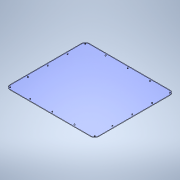
# Autodesk Inventor part: right_pane_outerl
Saved by Autodesk Inventor 2022 (Build 260153000, 153)
## iProperties
Created: 2021-05-16
Part Number: right_pane_outerl
Material: Generic
Document SubType Name: Modeling
Designer: gisen
Density: 1 g/cm^3
Appearance: Clear - Blue
Author: gisen
Autodesk Inventor part; units mm, degrees
ref_plane "YZ Plane" through (0, 0, 0) normal (1, 0, 0) x (0, 1, 0)
ref_plane "XZ Plane" through (0, 0, 0) normal (0, 1, 0) x (-1, 0, 0)
ref_plane "XY Plane" through (0, 0, 0) normal (0, 0, 1) x (1, 0, 0)
sketch "Sketch1" plane through (0, 0, 0) normal (0, 0, 1) x (1, 0, 0)
  line L0 (-196.0353, 191.75) -> (194.1012, 191.75)
  line L1 (213.9647, 171.6135) -> (213.9647, -172.019)
  line L2 (193.2337, -192.75) -> (-195.7732, -192.75)
  line L3 (-216.0353, -173.0121) -> (-216.0353, 171.75)
  line L4 (-205, 191.75) -> (205, -191.75) construction
  line L5 (205, 191.75) -> (-205, -191.75) construction
  arc A0 (-196.0353, 191.75) -> (-216.0353, 171.75) centre (-196.0353, 171.75) ccw
  arc A1 (-216.0353, -173.0121) -> (-195.7732, -192.75) centre (-196.0353, -172.75) ccw
  arc A2 (213.9647, 171.6135) -> (194.1012, 191.75) centre (193.9647, 171.75) ccw
  arc A3 (193.2337, -192.75) -> (213.9647, -172.019) centre (193.9647, -172.75) ccw
  point P0 (0, 0)
  dimension "d2" = 40
  dimension "d16" = 430
  dimension "d17" = 384.5
  dimension "d18" = 20
  dimension "d19" = 20
  dimension "d20" = 20
  dimension "d21" = 20
  dimension "d22" = 20
  dimension "d23" = 20
  constraints: 12 end point, 8 point on circle, 4 centre point, 2 horizontal, 2 midpoint, 2 parallel, 2 tangent, 1 perpendicular
  measures "d2" diameter of A0
  measures "d16" distance between parallel lines of L1 L3
  measures "d17" distance between parallel lines of L2 L0
  measures "d18" distance from line of L2 A1.centre
  measures "d19" distance from line of A1.centre L3
  measures "d20" distance from line of L1 A3.centre
  measures "d21" distance from line of A3.centre L2
  measures "d22" distance from line of A2.centre L0
  measures "d23" distance from line of A2.centre L1
extrude "Extrusion1" add sketch "Sketch1" along normal blind 3
sketch "Sketch2" plane through (0, 0, 3) normal (0, 0, 1) x (1, 0, 0)
  line L0 (194.1012, 191.75) -> (-196.0353, 191.75) projected
  arc A0 (-196.0353, 191.75) -> (-216.0353, 171.75) centre (-196.0353, 171.75) ccw projected
  line L1 (-216.0353, 171.75) -> (-216.0353, -173.0121) projected
  arc A1 (-216.0353, -173.0121) -> (-195.7732, -192.75) centre (-196.0353, -172.75) ccw projected
  line L2 (-195.7732, -192.75) -> (193.2337, -192.75) projected
  arc A2 (193.2337, -192.75) -> (213.9647, -172.019) centre (193.9647, -172.75) ccw projected
  line L3 (213.9647, -172.019) -> (213.9647, 171.6135) projected
  arc A3 (213.9647, 171.6135) -> (194.1012, 191.75) centre (193.9647, 171.75) ccw projected
  line L4 (-29.4365, -0.5) -> (27.4029, -0.5)
  line L5 (-1.0353, 26.0167) -> (-1.0353, -40.6326)
  point P0 (0, 0)
  point P1 (-206.0353, -182.75)
  point P2 (203.9647, -182.75)
  point P3 (-206.0353, 181.75)
  point P4 (203.9647, 181.75)
  dimension "d6" = 10
  dimension "d7" = 10
  dimension "d24" = 10
  dimension "d25" = 10
  dimension "d26" = 10
  dimension "d27" = 10
  dimension "d28" = 10
  dimension "d29" = 10
  constraints: 4 end point, 3 symmetric about line, 1 horizontal, 1 vertical
  measures "d6" distance from line of L2 point (-206.035, -182.75)
  measures "d7" distance from line of point (-206.035, -182.75) L1
  measures "d24" distance from line of L0 point (-206.035, 181.75)
  measures "d25" distance from line of L1 point (-206.035, 181.75)
  measures "d26" distance from line of L3 point (203.965, -182.75)
  measures "d27" distance from line of L2 point (203.965, -182.75)
  measures "d28" distance from line of L3 point (203.965, 181.75)
  measures "d29" distance from line of L0 point (203.965, 181.75)
hole "Hole1" at (-206.0353, -182.75, 3) at (203.9647, -182.75, 3) at (-206.0353, 181.75, 3) at (203.9647, 181.75, 3) direction (0, 0, -1) diameter 4.5 end through all
sketch "Sketch3" plane through (0, 0, 3) normal (0, 0, 1) x (1, 0, 0)
  line L0 (-195.7732, -192.75) -> (193.2337, -192.75) projected
  line L1 (-216.0353, 171.75) -> (-216.0353, -173.0121) projected
  line L2 (194.1012, 191.75) -> (-196.0353, 191.75) projected
  line L3 (213.9647, -172.019) -> (213.9647, 171.6135) projected
  line L4 (-112.0022, -0.2028) -> (58.7226, -0.2028)
  line L5 (-1.0353, -182.75) -> (-1.0353, -118.948)
  point P0 (0, 0)
  point P1 (-108.5353, -182.75)
  point P2 (-206.0353, -96.625)
  point P3 (-206.0353, 95.625)
  point P4 (-206.0353, -0.5)
  point P5 (106.4647, -182.75)
  point P6 (-108.5353, 182.3444)
  point P7 (106.4647, 182.3444)
  point P8 (-1.0353, 182.3444)
  point P9 (203.9647, -96.625)
  point P10 (203.9647, 95.625)
  point P11 (203.9647, -0.5)
  dimension "d30" = 10
  dimension "d31" = 10
  dimension "d38" = 384.5
  dimension "d41" = 288.375
  dimension "d42" = 192.25
  dimension "d43" = 96.125
  dimension "d44" = 430
  dimension "d45" = 107.5
  dimension "d46" = 215
  dimension "d47" = 322.5
  constraints: 6 symmetric about line, 4 end point, 1 horizontal, 1 vertical
  measures "d30" distance from line of L0 point (-108.535, -182.75)
  measures "d31" distance from line of L1 point (-206.035, -96.625)
  measures "d38" distance between parallel lines of L0 L2
  measures "d41" distance from line of point (-206.035, 95.625) L0
  measures "d42" distance from line of L0 point (-206.035, -0.5)
  measures "d43" distance from line of L0 point (-206.035, -96.625)
  measures "d44" distance between parallel lines of L3 L1
  measures "d45" distance from line of L1 point (-108.535, -182.75)
  measures "d46" distance from line of L1 L5.start
  measures "d47" distance from line of point (106.465, -182.75) L1
hole "Hole2" at (-108.5353, -182.75, 3) at (-206.0353, -96.625, 3) at (-206.0353, 95.625, 3) at (-206.0353, -0.5, 3) at (106.4647, -182.75, 3) at (-1.0353, -182.75, 3) at (-108.5353, 182.3444, 3) at (-1.0353, 182.3444, 3) at (106.4647, 182.3444, 3) at (203.9647, 95.625, 3) at (203.9647, -0.5, 3) at (203.9647, -96.625, 3) direction (0, 0, -1) diameter 4.5 end through all
equation "\"d22\" = d19"
equation "\"d23\" = d20"
equation "\"d26\" = d7"
equation "\"d41\" = 0.75 * d38"
equation "\"d42\" = 0.5 * d38"
equation "\"d43\" = 0.25 * d38"
equation "\"d45\" = 0.25 * d44"
equation "\"d46\" = 0.5 * d44"
equation "\"d47\" = 0.75 * d44"
body "Solid1"
